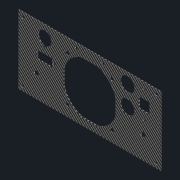
# Autodesk Inventor part: plate5
Saved by Autodesk Inventor 2021 (Build 250183000, 183)
## iProperties
Created: 2021-07-22
Part Number: plate5
Material: CFRP
Document SubType Name: Sheet Metal
Designer: yuta0
Density: 1.43 g/cm^3
Sheet Metal Rule: Default
Appearance: カーボンファイバー
Author: yuta0
Autodesk Inventor part; units mm, degrees
ref_plane "YZ Plane" through (0, 0, 0) normal (1, 0, 0) x (0, 1, 0)
ref_plane "XZ Plane" through (0, 0, 0) normal (0, 1, 0) x (-1, 0, 0)
ref_plane "XY Plane" through (0, 0, 0) normal (0, 0, 1) x (1, 0, 0)
sketch "スケッチ1" plane through (0, 0, 0) normal (0, 0, 1) x (1, 0, 0)
  line L0 (-80, -38.5) -> (80, -38.5)
  line L1 (80, -38.5) -> (80, 38.5)
  line L2 (80, 38.5) -> (-80, 38.5)
  line L3 (-80, 38.5) -> (-80, -38.5)
  line L4 (-80, -38.5) -> (80, 38.5) construction
  line L5 (80, -38.5) -> (-80, 38.5) construction
  point P0 (0, 0)
  dimension "d0" = 160
  dimension "d1" = 77
  measures "d0" distance of L2.end L1.end
  measures "d1" distance of L1.end L0.end
extrude "プレート1" add sketch "スケッチ1" along normal blind 1
sketch "スケッチ2" plane through (0, 0, 1) normal (0, 0, 1) x (1, 0, 0)
  line L0 (-80, -38.5) -> (-80, 38.5) projected
  line L1 (80, -38.5) -> (-80, -38.5) projected
  line L2 (80, 38.5) -> (80, -38.5) projected
  line L3 (-80, 38.5) -> (80, 38.5) projected
  line L4 (75, 33.5) -> (75, -33.5)
  line L5 (75, -33.5) -> (-75, -33.5)
  line L6 (-75, -33.5) -> (-75, 33.5)
  line L7 (-75, 33.5) -> (75, 33.5)
  point P0 (0, 0)
  dimension "d3" = 5
  constraints: 8 end point, 3 other
  measures "d3" distance between parallel lines of L3 L7
hole "穴1" at (-75, 33.5, 1) at (-75, -33.5, 1) at (75, -33.5, 1) at (75, 33.5, 1) direction (0, 0, -1) diameter 3.4 depth 1 clearance for "Flat Head Machine Screw" size "M3" standard "Ansi Metric M Profile"
sketch "スケッチ3" plane through (0, 0, 1) normal (0, 0, 1) x (1, 0, 0)
  line L0 (30, -31.5) -> (-30, -31.5) construction
  line L1 (-30, -31.5) -> (-30, 28.5) construction
  line L2 (-30, 28.5) -> (30, 28.5) construction
  line L3 (30, 28.5) -> (30, -31.5) construction
  line L4 (30, -31.5) -> (-30, 28.5) construction
  line L5 (-30, -31.5) -> (30, 28.5) construction
  line L6 (-69, -4.5) -> (-31.7, -4.5) construction
  line L7 (-31.7, -4.5) -> (-31.7, 15.5) construction
  line L8 (-31.7, 15.5) -> (-69, 15.5) construction
  line L9 (-69, -4.5) -> (-31.7, 15.5) construction
  line L10 (-31.7, -4.5) -> (-69, 15.5) construction
  circle A0 centre (42.5, 5) radius 9.6 construction
  line L11 (54, -3.5) -> (69, -3.5) construction
  line L12 (69, -3.5) -> (69, 35.5) construction
  line L13 (69, 35.5) -> (54, 35.5) construction
  line L14 (54, 35.5) -> (54, -3.5) construction
  line L15 (54, -3.5) -> (69, 35.5) construction
  line L16 (69, -3.5) -> (54, 35.5) construction
  line L17 (-80, 38.5) -> (80, 38.5) construction
  line L18 (80, 38.5) -> (80, -38.5) construction
  line L19 (-80, -38.5) -> (-80, 38.5) projected
  line L20 (80, -38.5) -> (-80, -38.5) projected
  line L21 (-58.6, 1) -> (-42.1, 1)
  line L22 (-42.1, 1) -> (-42.1, 10)
  line L23 (-42.1, 10) -> (-58.6, 10)
  line L24 (-58.6, 10) -> (-58.6, 1)
  line L25 (-58.6, 1) -> (-42.1, 10) construction
  line L26 (-42.1, 1) -> (-58.6, 10) construction
  line L27 (55.5, 10) -> (67.5, 10)
  line L28 (67.5, 10) -> (67.5, 22)
  line L29 (67.5, 22) -> (55.5, 22)
  line L30 (55.5, 22) -> (55.5, 10)
  line L31 (55.5, 10) -> (67.5, 22) construction
  line L32 (67.5, 10) -> (55.5, 22) construction
  circle A1 centre (0, -1.5) radius 30.5
  line L33 (-29, -30.5) -> (29, -30.5)
  line L34 (29, -30.5) -> (29, 27.5)
  line L35 (29, 27.5) -> (-29, 27.5)
  line L36 (-29, 27.5) -> (-29, -30.5)
  line L37 (-29, -30.5) -> (29, 27.5) construction
  line L38 (29, -30.5) -> (-29, 27.5) construction
  circle A2 centre (42.5, 5) radius 8.1
  line L39 (39.4406, 12.5) -> (45.5594, 12.5)
  arc A3 (-48.8573, 18.048) -> (-51.8427, 18.048) centre (-50.35, 25.5) ccw
  circle A4 centre (-50.35, 25.5) radius 10.5 construction
  arc A5 (-51.8427, 18.048) -> (-48.8573, 18.048) centre (-50.35, 17.9) ccw
  circle A6 centre (42.5, 27) radius 8.1
  circle A7 centre (42.5, 27) radius 9 construction
  line L40 (42.5, 16.0851) -> (52.1, 10.5426) construction
  line L41 (52.1, 10.5426) -> (52.1, -0.5426) construction
  line L42 (52.1, -0.5426) -> (42.5, -6.0851) construction
  line L43 (42.5, -6.0851) -> (32.9, -0.5426) construction
  line L44 (32.9, -0.5426) -> (32.9, 10.5426) construction
  line L45 (32.9, 10.5426) -> (42.5, 16.0851) construction
  circle A8 centre (42.5, 5) radius 11.0851 construction
  point P0 (-50.35, 5.5)
  point P1 (61.5, 16)
  point P2 (61.5, 16)
  point P3 (-50.35, 5.5)
  point P4 (-29, 7.9472)
  point P5 (-29, -10.9472)
  point P6 (-9.4472, -30.5)
  point P7 (9.4472, -30.5)
  point P8 (29, -10.9472)
  point P9 (29, 7.9472)
  point P10 (9.4472, 27.5)
  point P11 (-9.4472, 27.5)
  point P12 (61.5, 16)
  point P13 (-50.35, 5.5)
  point P14 (0, -1.5)
  point P15 (0, 0)
  dimension "d11" = 60
  dimension "d12" = 60
  dimension "d13" = 37.3
  dimension "d14" = 20
  dimension "d15" = 19.2
  dimension "d16" = 15
  dimension "d17" = 39
  dimension "d20" = 0
  dimension "d28" = 16.5
  dimension "d29" = 9
  dimension "d30" = 12
  dimension "d31" = 12
  dimension "d32" = 61
  dimension "d33" = 58
  dimension "d34" = 58
  dimension "d35" = 16.2
  dimension "d36" = 7.5
  dimension "d78" = 0
  dimension "d86" = 15.2
  dimension "d88" = 13
  dimension "d89" = 21
  dimension "d90" = 20
  dimension "d91" = 11
  dimension "d94" = 3
  dimension "d95" = 3
  dimension "d96" = 16.2
  dimension "d97" = 22
  dimension "d98" = 18
  dimension "d99" = 11
  dimension "d101" = 19.2
  dimension "d102" = 19
  dimension "d104" = 11
  dimension "d106" = 1.5
  constraints: 84 end point, 17 midpoint, 11 parallel, 8 centre point, 7 horizontal, 7 point on circle, 6 coincident, 6 perpendicular, 6 vertical alignment, 15 other
  measures "d11" distance of L1.end L2.end
  measures "d12" distance of L0.end L1.end
  measures "d13" distance of L8.end L7.end
  measures "d14" distance of L7.end L6.end
  measures "d15" diameter of A0
  measures "d16" distance of L13.end L12.end
  measures "d17" distance of L12.end L11.end
  measures "d20" distance of point (0, -1.5) point (0, -1.5)
  measures "d28" distance of L23.end L22.end
  measures "d29" distance of L22.end L21.end
  measures "d30" distance of L29.end L28.end
  measures "d31" distance of L28.end L27.end
  measures "d32" diameter of A1
  measures "d33" distance of L35.end L34.end
  measures "d34" distance of L34.end L33.end
  measures "d35" diameter of A2
  measures "d36" distance from line of A0.centre L39
  measures "d78" distance of point (0, -1.5) point (0, -1.5)
  measures "d86" diameter of A3
  measures "d88" distance from line of L17 A3.centre
  measures "d89" diameter of A4
  measures "d90" distance of A4.centre point (-50.35, 5.5)
  measures "d91" distance from line of L19 L8.end
  measures "d94" diameter of A5
  measures "d95" distance between parallel lines of L17 L13
  measures "d96" diameter of A6
  measures "d97" distance of A0.centre A6.centre
  measures "d98" diameter of A7
  measures "d99" vertical distance of point (61.5, 16) A6.centre
  measures "d101" distance between parallel lines of L43 L40
  measures "d102" horizontal distance of A6.centre point (61.5, 16)
  measures "d104" distance between parallel lines of L18 L12
  measures "d106" distance of point (0, 0) point (0, -1.5)
extrude "押し出し1" cut sketch "スケッチ3" against normal blind 16.2 contours L24 L23 L22 L21 | L30 L29 L28 L27 | L34 A1 L33 L36 L35 | A2 L39 | A5 A3 | A6 picked at (42.2004, 7.3167)
sketch "スケッチ4" plane through (0, 0, 1) normal (0, 0, 1) x (1, 0, 0)
  arc A0 (-9.4472, 27.5) -> (-29, 7.9472) centre (0, -1.5) ccw projected
  line L0 (-25, -26.5) -> (25, -26.5)
  line L1 (25, -26.5) -> (25, 23.5)
  line L2 (25, 23.5) -> (-25, 23.5)
  line L3 (-25, 23.5) -> (-25, -26.5)
  line L4 (-25, -26.5) -> (25, 23.5) construction
  line L5 (25, -26.5) -> (-25, 23.5) construction
  point P0 (0, 0)
  dimension "d39" = 50
  dimension "d40" = 50
  constraints: 12 end point, 2 midpoint, 2 parallel, 1 horizontal, 1 perpendicular
  measures "d39" distance of L2.end L1.end
  measures "d40" distance of L1.end L0.end
hole "穴2" at (-25, 23.5, 1) at (25, 23.5, 1) at (25, -26.5, 1) at (-25, -26.5, 1) direction (0, 0, -1) diameter 4.5 end through all clearance for "Socket Head Cap Screw" size "M4" standard "Ansi Metric M Profile"
sketch "スケッチ5" plane through (0, 0, 1) normal (0, 0, 1) x (1, 0, 0)
  line L0 (-58.6, 1) -> (-58.6, 10) projected
  line L1 (-58.6, 10) -> (-42.1, 10) projected
  line L2 (-42.1, 1) -> (-58.6, 1) projected
  line L3 (-42.1, 10) -> (-42.1, 1) projected
  line L4 (-42.1, 1) -> (-58.6, 1)
  line L5 (-58.6, 1) -> (-58.6, 10)
  line L6 (-58.6, 10) -> (-42.1, 10)
  line L7 (-42.1, 10) -> (-42.1, 1)
  line L8 (-42.1, 1) -> (-58.6, 10) construction
  line L9 (-58.6, 1) -> (-42.1, 10) construction
  line L10 (67.5, 10) -> (55.5, 10)
  line L11 (55.5, 10) -> (55.5, 22)
  line L12 (55.5, 22) -> (67.5, 22)
  line L13 (67.5, 22) -> (67.5, 10)
  line L14 (67.5, 10) -> (55.5, 22) construction
  line L15 (55.5, 10) -> (67.5, 22) construction
  point P0 (0, 0)
  point P1 (-40.05, 5.5)
  point P2 (-60.65, 5.5)
  point P3 (-50.35, 5.5)
  point P4 (-50.35, 5.5)
  point P5 (-50.35, 5.5)
  point P6 (61.5, 31)
  point P7 (61.5, 1)
  point P8 (61.5, 16)
  point P9 (61.5, 16)
  point P10 (61.5, 16)
  dimension "d48" = 10.3
  dimension "d49" = 10.3
  dimension "d76" = 15
  dimension "d77" = 15
  constraints: 24 end point, 8 midpoint, 4 parallel, 2 coincident, 2 horizontal, 2 horizontal alignment, 2 perpendicular, 2 vertical alignment
  measures "d48" distance of point (-50.35, 5.5) point (-40.05, 5.5)
  measures "d49" distance of point (-60.65, 5.5) point (-50.35, 5.5)
  measures "d76" distance of point (61.5, 31) point (61.5, 16)
  measures "d77" distance of point (61.5, 1) point (61.5, 16)
hole "穴3" at (-40.05, 5.5, 1) at (-60.65, 5.5, 1) at (61.5, 1, 1) at (61.5, 31, 1) direction (0, 0, -1) diameter 2.9 end through all clearance for "Socket Head Cap Screw" size "M2.5" standard "Ansi Metric M Profile"
fillet "コーナーR1" radius 1 8 edges at (55.5, 22, 0.5) (67.5, 22, 0.5) (67.5, 10, 0.5) (55.5, 10, 0.5) (-58.6, 10, 0.5) (-58.6, 1, 0.5) (-42.1, 1, 0.5) (-42.1, 10, 0.5)
fillet "コーナーR2" radius 5 8 edges at (-29, -10.9472, 0.5) (-9.4472, -30.5, 0.5) (9.4472, -30.5, 0.5) (29, -10.9472, 0.5) (29, 7.9472, 0.5) (9.4472, 27.5, 0.5) (-9.4472, 27.5, 0.5) (-29, 7.9472, 0.5)
sketch "スケッチ6" plane through (0, 0, 1) normal (0, 0, 1) x (1, 0, 0)
  line L0 (80, -38.5) -> (-80, -38.5) projected
  point P0 (0, 0)
  point P1 (-60, -13.5)
  point P2 (60, -13.5)
  dimension "d62" = 25
  dimension "d63" = 60
  dimension "d64" = 60
  constraints: 1 horizontal alignment
  measures "d62" distance from line of L0 point (-60, -13.5)
  measures "d63" horizontal distance of point (0, 0) point (-60, -13.5)
  measures "d64" horizontal distance of point (60, -13.5) point (0, 0)
hole "穴4" at (-60, -13.5, 1) at (60, -13.5, 1) direction (0, 0, -1) diameter 5.5 end through all clearance for "Flat Head Machine Screw" size "M5" standard "Ansi Metric M Profile"
fillet "コーナーR3" radius 2 2 edges at (39.4406, 12.5, 0.5) (45.5594, 12.5, 0.5)
fillet "コーナーR4" radius 1.5 2 edges at (-51.8427, 18.048, 0.5) (-48.8573, 18.048, 0.5)
sketch "スケッチ7" plane through (0, 0, 0) normal (0, 0, -1) x (-1, 0, 0)
  line L0 (-80, 38.5) -> (80, 38.5) projected
  point P0 (0, 0)
  point P1 (-15, 33.5)
  point P2 (15, 33.5)
  dimension "d107" = 30
  dimension "d108" = 5
  dimension "d109" = 15
  constraints: 1 horizontal alignment
  measures "d107" distance of point (-15, 33.5) point (15, 33.5)
  measures "d108" distance from line of L0 point (15, 33.5)
  measures "d109" horizontal distance of point (0, 0) point (15, 33.5)
hole "穴5" at (15, 33.5, 0) at (-15, 33.5, 0) direction (0, 0, 1) diameter 3.4 end through all clearance for "Flat Head Machine Screw" size "M3" standard "Ansi Metric M Profile"
equation "\"d9\" = Thickness"
equation "\"d46\" = Thickness"
equation "\"d49\" = d48"
equation "\"d77\" = d76"
equation "\"d55\" = Thickness"
equation "\"d70\" = Thickness"
equation "\"d2\" = Thickness"
equation "\"BendRadius\" = Thickness"
equation "\"BendReliefWidth\" = Thickness"
equation "\"BendReliefDepth\" = 0.5 * Thickness"
equation "\"CornerReliefSize\" = 4 * Thickness"
equation "\"MinimumRemnant\" = 2 * Thickness"
equation "\"TransitionRadius\" = BendRadius"
equation "\"JacobiRadiusSize\" = Thickness"
equation "\"GapSize\" = Thickness"
equation "\"Thickness\" = 1"
